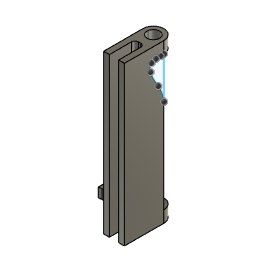
Fwd_Flap (Autodesk Fusion 360 design; units mm, degrees)
Autodesk Fusion 360 part; units mm, degrees
sketch "Sketch1" plane through (0, 0, 0) normal (0, 0, 1) x (1, 0, 0)
  line L0 (-3.8994, -6.1193, 0.219) -> (-3.8994, -13.1193, 0.219)
  line L1 (4.3847, -1.0062, 0.219) -> (4.3847, -6.0062, 0.219)
  line L2 (-3.8994, -1.1193, 0.219) -> (-3.8994, -6.1193, 0.219)
  line L3 (4.3847, -6.0062, 0.219) -> (4.3847, -13.0062, 0.219)
  circle A0 through (11.3847, -3.5062, 0.219) (9.8847, -2.6401, 0.219) (9.8847, -4.3722, 0.219)
  line L4 (13.8847, -6.0738, 0.219) -> (12.3847, -6.0062, 0.219)
  line L5 (-11.8994, -1.1193, 0.219) -> (-3.8994, -1.1193, 0.219)
  line L6 (12.3847, -1.0062, 0.219) -> (13.8847, -1.0062, 0.219)
  line L7 (12.3847, -6.0062, 0.219) -> (12.3847, -1.0062, 0.219)
  arc A1 through (-3.8994, -13.1193, 0.219) (-5.9497, -8.1696, 0.219) (-10.8994, -6.1193, 0.219)
  line L8 (-13.3994, -6.2991, 0.219) -> (-11.8994, -6.1193, 0.219)
  line L9 (-13.3994, -1.1193, 0.219) -> (-13.3994, -6.2991, 0.219)
  circle A2 through (-8.8994, -3.6193, 0.219) (-10.3994, -2.7533, 0.219) (-10.3994, -4.4854, 0.219)
  line L10 (-11.8994, -1.1193, 0.219) -> (-13.3994, -1.1193, 0.219)
  line L11 (13.8847, -1.0062, 0.219) -> (13.8847, -6.0738, 0.219)
  line L12 (-10.8994, -6.1193, 0.219) -> (-11.8994, -6.1193, 0.219)
  line L13 (11.3847, -6.0062, 0.219) -> (12.3847, -6.0062, 0.219)
  line L14 (12.3847, -1.0062, 0.219) -> (4.3847, -1.0062, 0.219)
  line L15 (-11.8994, -6.1193, 0.219) -> (-11.8994, -1.1193, 0.219)
  arc A3 through (11.3847, -6.0062, 0.219) (6.4349, -8.0564, 0.219) (4.3847, -13.0062, 0.219)
  line L16 (0.498, 0) -> (0.498, 3.4859)
  circle A4 centre (0.498, 3.4859) radius 2.7
  circle A5 centre (0.498, 3.4859) radius 4.5
  line L17 (-4.002, 3.4747) -> (4.998, 3.4747)
  line L18 (4.998, 3.4747) -> (4.9559, -13.4145)
  line L19 (-4.002, 3.4747) -> (-4.002, -13.3921)
  line L20 (-4.002, -13.3921) -> (4.9559, -13.4145)
  line L21 (0.498, 0) -> (0.498, -2.4014)
  line L22 (0.498, -2.4014) -> (0.9942, -2.4014)
  line L23 (2.498, -2.4014) -> (0.498, -2.4014)
  line L24 (0.498, -2.4014) -> (-0.0057, -2.4014)
  line L25 (-1.5057, -3.8976) -> (-1.5294, -13.3983)
  line L26 (2.4942, -3.9051) -> (2.4705, -13.4083)
  arc A6 (-0.0057, -2.4014) -> (-1.5057, -3.8976) centre (-0.0057, -3.9014) ccw
  arc A7 (2.4942, -3.9051) -> (0.9942, -2.4014) centre (0.9942, -3.9014) ccw
  point P0 (-0.003, 2.4938)
  point P1 (-0.003, -7.2965)
  point P2 (0.498, 0)
  point P3 (-0.1153, 2.4938)
  point P4 (-1.502, -2.4014)
  dimension "d49" = 5
  dimension "d51" = 8
  dimension "d52" = 2
  dimension "d53" = 6
  dimension "d54" = 2.5
  dimension "d55" = 7
  dimension "d56" = 1.5
  dimension "d57" = 1.5
  dimension "d11" = 9
  dimension "d12" = 5.4
  dimension "d13" = 2
  dimension "d14" = 2
  dimension "d15" = 1.5
  dimension "d16" = 1.5
  constraint coincident P2 L16.start
  constraint vertical L16
  constraint coincident L16.end A4.centre
  constraint concentric A4 A5
  constraint coincident A5 L17.start
  constraint coincident A5 L17.end
  constraint tangent A5 L18
  constraint perpendicular L17 L19
  constraint perpendicular L18 L20
  constraint parallel L16 L21
  constraint perpendicular L21 L22
  constraint perpendicular L21 L24
  constraint coincident L20 L25.end
  constraint perpendicular L20 L25
  constraint coincident L20 L26.end
  constraint perpendicular L20 L26
  constraint coincident P4 L24
  constraint coincident P4 L25
  constraint tangent L24 A6
  constraint tangent L25 A6
  constraint coincident L23.start L26
  constraint coincident L23.start L22
  constraint tangent L26 A7
  constraint tangent L22 A7
  measures "d11" diameter of A5
  measures "d12" diameter of A4
  measures "d13" distance of L21.end P4
  measures "d14" distance of L21.end L23.start
  measures "d15" radius of A6
  measures "d16" radius of A7
extrude "Extrude1" add sketch "Sketch1" along normal blind 68 contours L16 A4 A5 L17 L21 | L16 A4 A5 L17 L21 | A5 L19 L20 L21 L24 L25 A6 | A5 L18 L20 L21 L22 L23 L26 A7
extrude "Extrude2" add sketch "Sketch1" along normal blind 5 contours A4 A5 L17
extrude "Extrude3" add sketch "Sketch1" along normal blind 5 from surface at 63 contours A4 A5 L17
extrude "Extrude4" add sketch "Sketch1" along normal blind 4 from surface at 5 contours L0 L2 L5 A1 L12 L15 | L8 L9 L10 L15 in plane through (0, 0, 0.219) normal (0, 0, 1)
ref_plane "WorkPlane1" through (4.9769, -4.9699, 34) normal (0.999997, -0.002493, 0) x (0.002493, 0.999997, 0)
sketch "Sketch2" plane through (4.9769, -4.9699, 34) normal (0.999997, -0.002493, 0) x (0.002493, 0.999997, 0)
  spline S0 degree 5 poles (8.5256, 29.005) (8.4529, 29.0037) (8.304, 29.0016) (8.0699, 28.9996) (7.7363, 28.9992) (7.284, 29.0025) (6.7976, 29.0087) (6.2798, 29.0166) (5.7359, 29.0227) (5.1752, 29.0182) (4.6118, 28.987) (4.0671, 28.9018) (3.5665, 28.7292) (3.1369, 28.4389) (2.8023, 28.0105) (2.5808, 27.4428) (2.4842, 26.7495) (2.5174, 25.9536) (2.679, 25.082) (2.9604, 24.1597) (3.3463, 23.205) (3.8162, 22.2311) (4.3464, 21.2466) (4.9117, 20.2566) (5.4869, 19.2638) (6.0491, 18.2689) (6.5786, 17.2719) (7.0613, 16.2728) (7.4875, 15.2716) (7.8512, 14.2683) (8.1489, 13.2629) (8.3333, 12.457) (8.4413, 11.8516) (8.4998, 11.4476) (8.5256, 11.2455) knots 0 0 0 0 0 0 0.033333 0.066667 0.1 0.133333 0.166667 0.2 0.233333 0.266667 0.3 0.333333 0.366667 0.4 0.433333 0.466667 0.5 0.533333 0.566667 0.6 0.633333 0.666667 0.7 0.733333 0.766667 0.8 0.833333 0.866667 0.9 0.933333 0.966667 1 1 1 1 1 1
  line L0 (8.5256, 11.2455) -> (8.5256, 29.005)
  point P0 (7.1122, 29.005)
  point P1 (5.022, 29.005)
  point P2 (3.105, 28.3495)
  point P3 (2.6845, 25.171)
  point P4 (6.0336, 18.2818)
  constraint vertical L0
extrude "Extrude5" cut sketch "Sketch2" against normal blind 10
